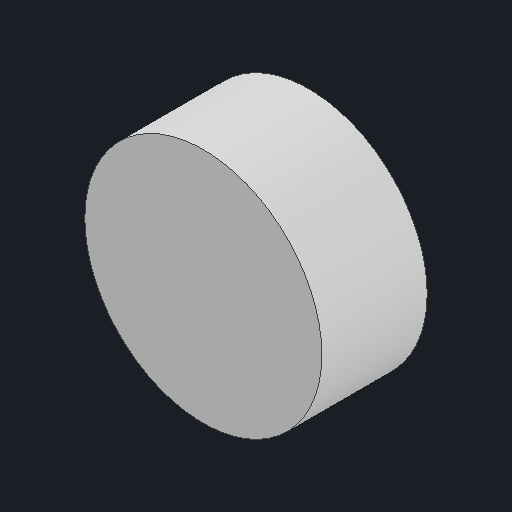
# Autodesk Inventor part: Part24
Saved by Autodesk Inventor 2027.1 (Build 311270010, 270A)
## iProperties
Created: 2026-09-29
Part Number: Part24
Material: Generic
Document SubType Name: Modeling
Designer: daniel
Density: 1 g/cm^3
Appearance: Default
Author: daniel
Autodesk Inventor part; units mm, degrees
ref_plane "YZ Plane" through (0, 0, 0) normal (1, 0, 0) x (0, 1, 0)
ref_plane "XZ Plane" through (0, 0, 0) normal (0, 1, 0) x (-1, 0, 0)
ref_plane "XY Plane" through (0, 0, 0) normal (0, 0, 1) x (1, 0, 0)
sketch "Sketch1" plane through (0, 0, 0) normal (0, 0, 1) x (1, 0, 0)
  circle A0 centre (0, 0) radius 22.5
  dimension "d0" = 45
  constraints: 1 centre point, 1 coincident
  measures "d0" diameter of A0
extrude "Extrusion1" add sketch "Sketch1" along normal blind 20
equation "\"d1\" = ProductLedHeight"
equation "\"ProductLedHeight\" = 20"
equation "\"GridProcutClearance\" = 3"
equation "\"GridBorderThickness\" = 5"
equation "\"GridBorderFillets\" = 7"
equation "\"GridTotalSize\" = 63"
equation "\"BaseTotalWidth\" = 652"
equation "\"WorkspaceLength\" = 652"
equation "\"AxesBaseFillet\" = 15"
equation "\"WorkspaceWidth\" = 372"
equation "\"ProductTotalHeight\" = 45"
equation "\"VerticalStroke\" = 85"
equation "\"Zaxis\" = 223"
equation "\"WorkspaceHeight\" = 166.5"
equation "\"BaseTotalLength\" = 912"
equation "\"DistanceBetweenGrid\" = 5"
equation "\"CylinderStroke\" = 75"
body "Solid1"
